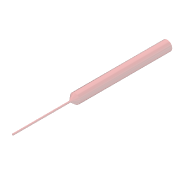
# Autodesk Inventor part: cellSTORM_laserbeam_meander
Saved by Autodesk Inventor 2019.4 (Build 234330000, 330)
## iProperties
Created: 2020-04-17
Part Number: cellSTORM_laserbeam_meander
Material: Generic
Document SubType Name: Modeling
Designer: diederichbenedict
Density: 1 g/cm^3
Appearance: Polycarbonate - Clear
Author: diederichbenedict
Autodesk Inventor part; units mm, degrees
ref_plane "YZ Plane" through (0, 0, 0) normal (1, 0, 0) x (0, 1, 0)
ref_plane "XZ Plane" through (0, 0, 0) normal (0, 1, 0) x (-1, 0, 0)
ref_plane "XY Plane" through (0, 0, 0) normal (0, 0, 1) x (1, 0, 0)
sketch "Sketch1" plane through (0, 0, 0) normal (0, 0, 1) x (1, 0, 0)
  circle A0 centre (0, 0) radius 6 projected
  circle A1 centre (0, 0) radius 2
  point P0 (0, 0)
  dimension "d0" = 4
  constraints: 1 centre point
  measures "d0" radial gap between concentric circles of A0 A1
ref_plane "Work Plane1" through (-3.5125, -3.5125, 37.5) normal (0, 0, 1) x (0.9086751, 0.417504, 0)
extrude "Extrusion1" add sketch "Sketch1" along normal up to surface (37.5 mm away) contours A1
sketch "Sketch2" plane through (0, 0, 37.5) normal (0, 0, 1) x (1, 0, 0)
  circle A0 centre (0, 0) radius 2 projected
  point P0 (0, 0)
extrude "Extrusion2" add sketch "Sketch2" along normal blind 2 draft -40
sketch "Sketch3" plane through (0, 0, 39.5) normal (0, 0, 1) x (1, 0, 0)
  circle A0 centre (0, 0) radius 0.3218 projected
  point P0 (0, 0)
ref_plane "Work Plane2" through (-0.9, -20.4499, 62.8) normal (0, 0, 1) x (1, 0, 0)
extrude "Extrusion3" add sketch "Sketch3" along normal up to surface (23.3 mm away)
body "Solid1"
